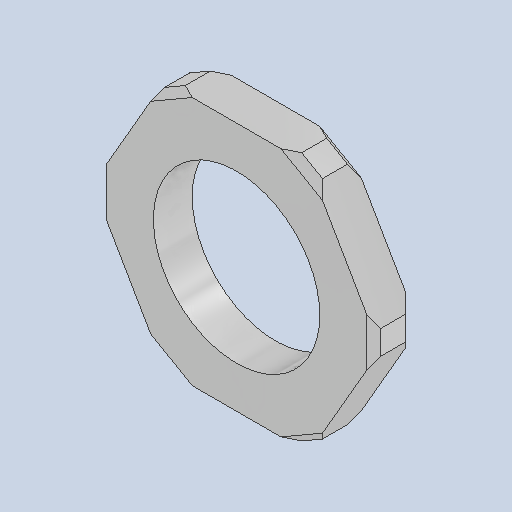
# Autodesk Inventor part: c-t4140012051-000-a-3d_NUT
Saved by Autodesk Inventor 2024.2 (Build 282272000, 272)
## iProperties
Created: 2020-06-14
Part Number: c-t4140012051-000-a-3d_NUT
Material: Generic
Document SubType Name: Modeling
Designer: Viktor Lindström
Density: 1 g/cm^3
Appearance: Default
Author: Viktor Lindström
Autodesk Inventor part; units mm, degrees
ref_plane "YZ Plane" through (0, 0, 0) normal (1, 0, 0) x (0, 1, 0)
ref_plane "XZ Plane" through (0, 0, 0) normal (0, 1, 0) x (-1, 0, 0)
ref_plane "XY Plane" through (0, 0, 0) normal (0, 0, 1) x (1, 0, 0)
sketch "Sketch1" plane through (0, 0, 0) normal (0, 0, 1) x (1, 0, 0)
  line L0 (10.3923, 0) -> (5.1962, -9)
  line L1 (5.1962, -9) -> (-5.1962, -9)
  line L2 (-5.1962, -9) -> (-10.3923, 0)
  line L3 (-10.3923, 0) -> (-5.1962, 9)
  line L4 (-5.1962, 9) -> (5.1962, 9)
  line L5 (5.1962, 9) -> (10.3923, 0)
  point P0 (0, 0)
  point P1 (0, 0)
  dimension "d0" = 18
  constraints: 12 end point, 1 coincident, 13 other
  measures "d0" distance between parallel lines of L1 L4
extrude "Extrusion1" add sketch "Sketch1" along normal blind 2.8
sketch "Sketch2" plane through (0, 0, 2.8) normal (0, 0, 1) x (1, 0, 0)
  circle A0 centre (0, 0) radius 6
  dimension "d3" = 12
  constraints: 1 centre point, 1 coincident
  measures "d3" diameter of A0
extrude "Extrusion2" cut sketch "Sketch2" against normal through all
chamfer "Chamfer1" distance 1 angle 45 6 edges at (5.1962, 9, 1.4) (-5.1962, 9, 1.4) (10.3923, 0, 1.4) (5.1962, -9, 1.4) (-5.1962, -9, 1.4) (-10.3923, 0, 1.4)
chamfer "Chamfer2" distance 0.5 angle 45 12 edges at (-9.8923, 0, 2.8) (-4.9462, -8.567, 2.8) (4.9462, -8.567, 2.8) (9.8923, 0, 2.8) (4.9462, 8.567, 2.8) (-4.9462, 8.567, 2.8) (-4.9462, 8.567, 0) (-9.8923, 0, 0) (-4.9462, -8.567, 0) (4.9462, -8.567, 0) (9.8923, 0, 0) (4.9462, 8.567, 0)
body "Solid1"
